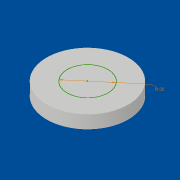
# Autodesk Inventor part: 941-printer calibration
Saved by Autodesk Inventor 2018 (Build 220112000, 112)
## iProperties
Created: 2020-12-26
Part Number: 941-printer calibration
Material: Generic
Document SubType Name: Modeling
Designer: Bunny320
Density: 1 g/cm^3
Appearance: Default
Author: Bunny320
Autodesk Inventor part; units mm, degrees
ref_plane "YZ Plane" through (0, 0, 0) normal (1, 0, 0) x (0, 1, 0)
ref_plane "XZ Plane" through (0, 0, 0) normal (0, 1, 0) x (-1, 0, 0)
ref_plane "XY Plane" through (0, 0, 0) normal (0, 0, 1) x (1, 0, 0)
sketch "Sketch1" plane through (0, 0, 0) normal (0, 0, 1) x (1, 0, 0)
  circle A0 centre (0, 0) radius 35
  dimension "d0" = 70
  constraints: 1 centre point, 1 coincident
  measures "d0" diameter of A0
extrude "Extrusion1" add sketch "Sketch1" along normal blind 11
sketch "Sketch2" plane through (0, 0, 11) normal (0, 0, 1) x (1, 0, 0)
  circle A0 centre (0, 0) radius 17.5
  dimension "d3" = 35
  constraints: 1 centre point, 1 coincident
  measures "d3" diameter of A0
equation "\"d0\" = bearing_61814_inner"
equation "\"d3\" = bearing_61807_inner"
equation "\"bearing_61807_inner\" = 35"
equation "\"bearing_61807_outer\" = 47.1"
equation "\"bearing_61814_inner\" = 70"
equation "\"bearing_61814_outer\" = 90.1"
equation "\"bearing_61705_outer\" = 32.1"
equation "\"bearing_61705_inner\" = 25"
equation "\"bearing_606_outer\" = 17.1"
equation "\"M3_adjustable\" = 3.2"
equation "\"gearbox_35_outer\" = 32.3"
equation "\"gearbox_42_outer\" = 42.3"
body "Solid1"
